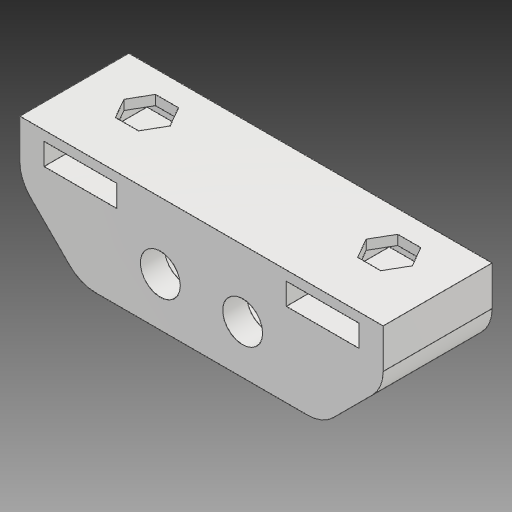
# Autodesk Inventor part: Kickerboard Winkel
Saved by Autodesk Inventor 2019.4 (Build 234330000, 330)
## iProperties
Part Number: Kickerboard Winkel
Material: PC/ABS-Kunststoff
Document SubType Name: Modeling
Designer: rYan
Density: 0.357273 g/cm^3
Appearance: Glatt - Weiß
Mass: 0.52583 g
Surface Area: 17.6014 cm^2
Volume: 1.47179 cm^3
Author: rYan
Autodesk Inventor part; units mm, degrees
ref_plane "YZ Plane" through (0, 0, 0) normal (1, 0, 0) x (0, 1, 0)
ref_plane "XZ Plane" through (0, 0, 0) normal (0, 1, 0) x (-1, 0, 0)
ref_plane "XY Plane" through (0, 0, 0) normal (0, 0, 1) x (1, 0, 0)
sketch "Skizze1" plane through (0, 0, 0) normal (1, 0, 0) x (0, 1, 0)
  line L0 (0, 0) -> (9, 0)
  line L1 (9, 0) -> (9, 9.5)
  line L2 (9, 9.5) -> (0, 9.5)
  line L3 (0, 9.5) -> (0, 0)
  dimension "d0" = 9
  dimension "d1" = 9.5
  constraints: 8 end point, 2 parallel, 1 horizontal, 1 perpendicular
  measures "d0" distance of L2.end L1.end
  measures "d1" distance of L1.end L0.end
extrude "Extrusion1" add sketch "Skizze1" along normal mid plane 30
sketch "Skizze2" plane through (-15, 0, 9.5) normal (0, 0, 1) x (1, 0, 0)
  line L0 (0, 0) -> (30, 0) projected
  line L1 (30, 9) -> (30, 0) projected
  line L2 (0, 9) -> (30, 9) projected
  line L3 (0, 0) -> (0, 9) projected
  line L4 (0, 5.5) -> (30, 5.5) construction
  line L5 (15, 0) -> (15, 9) construction
  point P0 (5, 5.5)
  point P1 (25, 5.5)
  dimension "d4" = 20
  dimension "d38" = 5.5
  constraints: 4 end point, 4 point on line, 1 midpoint, 1 perpendicular, 1 symmetric about line
  measures "d4" distance of point (25, 5.5) point (5, 5.5)
  measures "d38" distance between parallel lines of L4 L0
hole "Bohrung1" at (-10, 5.5, 9.5) at (10, 5.5, 9.5) direction (0, 0, -1) diameter 3.3 end through all
sketch "Skizze3" plane through (-15, 0, 0) normal (0, -1, 0) x (1, 0, 0)
  line L0 (30, 0) -> (0, 0) projected
  line L1 (30, 9.5) -> (30, 0) projected
  line L2 (0, 9.5) -> (30, 9.5) projected
  line L3 (0, 0) -> (0, 9.5) projected
  line L4 (0, 9.5) -> (0, 0) construction
  line L5 (0, 4) -> (30, 4) construction
  line L6 (30, 0) -> (30, 9.5) construction
  line L7 (15, 0) -> (15, 9.5) construction
  point P0 (11.6, 4)
  point P1 (18.4, 4)
  dimension "d13" = 6.8
  dimension "d14" = 5.5
  constraints: 4 end point, 4 point on line, 1 midpoint, 1 perpendicular, 1 symmetric about line
  measures "d13" distance of point (18.4, 4) point (11.6, 4)
  measures "d14" distance between parallel lines of L2 L5
hole "Bohrung2" at (-3.4, 0, 4) at (3.4, 0, 4) direction (0, 1, 0) diameter 3.3 end through all
sketch "Skizze5" plane through (-15, 0, 2.5) normal (0, -1, 0) x (1, 0, 0)
  line L0 (6.65, -2.5) -> (3.35, -2.5) projected
  line L1 (3.35, 7) -> (6.65, 7) projected
  line L2 (26.65, -2.5) -> (23.35, -2.5) projected
  line L3 (23.35, 7) -> (26.65, 7) projected
  line L4 (5, -2.5) -> (5, 7) construction
  line L5 (0, 7) -> (30, 7) construction
  line L6 (23.35, 7) -> (26.65, 7) construction
  line L7 (25, 7) -> (25, -2.5) construction
  line L8 (26.65, -2.5) -> (23.35, -2.5) construction
  line L9 (15, -2.5) -> (15, 7) construction
  line L10 (0, 7) -> (30, 7) construction
  line L11 (2, 4.4) -> (8, 4.4)
  line L12 (8, 4.4) -> (8, 6.2)
  line L13 (8, 6.2) -> (2, 6.2)
  line L14 (2, 6.2) -> (2, 4.4)
  line L15 (2, 4.4) -> (8, 6.2) construction
  line L16 (8, 4.4) -> (2, 6.2) construction
  line L17 (22, 4.4) -> (28, 4.4)
  line L18 (28, 4.4) -> (28, 6.2)
  line L19 (28, 6.2) -> (22, 6.2)
  line L20 (22, 6.2) -> (22, 4.4)
  line L21 (22, 4.4) -> (28, 6.2) construction
  line L22 (28, 4.4) -> (22, 6.2) construction
  point P0 (5, 5.3)
  point P1 (25, 5.3)
  dimension "d27" = 6
  dimension "d28" = 1.8
  dimension "d30" = 0.8
  constraints: 30 end point, 7 midpoint, 4 parallel, 3 perpendicular, 3 point on line, 2 horizontal, 5 other
  measures "d27" distance of L13.end L12.end
  measures "d28" distance of L12.end L11.end
  measures "d30" distance between parallel lines of L13 L1
extrude "Extrusion3" cut sketch "Skizze5" against normal blind 8.5
chamfer "Fase1" distance 5 angle 45 2 edges at (15, 4.5, 0) (-15, 4.5, 0)
fillet "Rundung1" radius 3 6 edges at (-15, 4.5, 5) (15, 4.5, 5) (-10, 8.075, 0) (-10, 1.925, 0) (10, 8.075, 0) (10, 1.925, 0)
sketch "Skizze6" plane through (-15, 9, 9.5) normal (0, 1, 0) x (1, 0, 0)
  circle A0 centre (18.4, 5.5) radius 1.65 projected
  circle A1 centre (11.6, 5.5) radius 1.65 projected
  line L0 (18.4, 5.5) -> (11.6, 5.5) construction
  line L1 (18.4, 8.6) -> (11.6, 8.6)
  line L2 (11.6, 2.4) -> (18.4, 2.4)
  arc A2 (18.4, 2.4) -> (18.4, 8.6) centre (18.4, 5.5) ccw
  arc A3 (11.6, 8.6) -> (11.6, 2.4) centre (11.6, 5.5) ccw
  point P0 (15, 9.5)
  point P1 (15, 5.5)
  dimension "d39" = 6.2
  constraints: 8 end point, 4 point on circle, 4 tangent, 2 centre point, 1 horizontal, 1 midpoint, 1 parallel
  measures "d39" diameter of A3
extrude "Extrusion4" cut sketch "Skizze6" against normal blind 7
sketch "Skizze7" plane through (-15, 0, 9.5) normal (0, 0, 1) x (1, 0, 0)
  circle A0 centre (5, 5.5) radius 1.65 projected
  circle A1 centre (25, 5.5) radius 1.65 projected
  line L0 (5.9526, 3.85) -> (4.0474, 3.85)
  line L1 (4.0474, 3.85) -> (3.0947, 5.5)
  line L2 (3.0947, 5.5) -> (4.0474, 7.15)
  line L3 (4.0474, 7.15) -> (5.9526, 7.15)
  line L4 (5.9526, 7.15) -> (6.9053, 5.5)
  line L5 (6.9053, 5.5) -> (5.9526, 3.85)
  circle A2 centre (25, 5.5) radius 1.65 projected
  line L6 (24.0474, 3.85) -> (23.0947, 5.5)
  line L7 (23.0947, 5.5) -> (24.0474, 7.15)
  line L8 (24.0474, 7.15) -> (25.9526, 7.15)
  line L9 (25.9526, 7.15) -> (26.9053, 5.5)
  line L10 (26.9053, 5.5) -> (25.9526, 3.85)
  line L11 (25.9526, 3.85) -> (24.0474, 3.85)
  point P0 (15, 0)
  constraints: 24 end point, 2 coincident, 2 horizontal, 2 tangent, 26 other
extrude "Extrusion5" cut sketch "Skizze7" against normal through all contours A0 L4 L5 | A0 L3 L4 | L5 L0 A0 | A0 L2 L3 | L0 L1 A0 | A0 L1 L2 | A1 L9 L10 | A1 L8 L9 | L10 L11 A1 | A1 L7 L8 | L11 L6 A1 | A1 L6 L7
